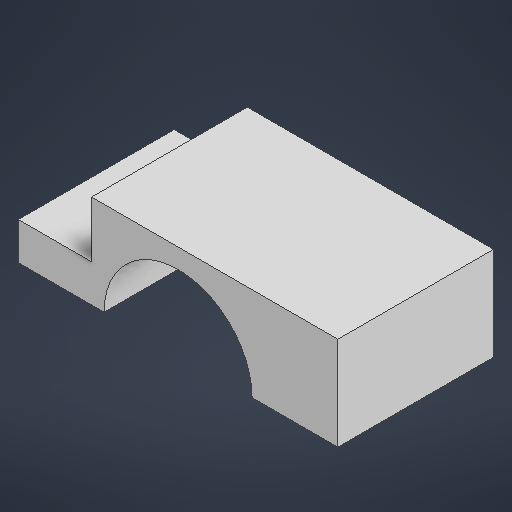
# Autodesk Inventor part: dg_clamp
Saved by Autodesk Inventor 2026.1 (Build 301233020, 233B)
## iProperties
Created: 2026-03-05
Part Number: dg_clamp
Material: Generic
Document SubType Name: Modeling
Designer: Dylan
Density: 1 g/cm^3
Appearance: Default
Author: Dylan
Autodesk Inventor part; units mm, degrees
ref_plane "YZ Plane" through (0, 0, 0) normal (1, 0, 0) x (0, 1, 0)
ref_plane "XZ Plane" through (0, 0, 0) normal (0, 1, 0) x (-1, 0, 0)
ref_plane "XY Plane" through (0, 0, 0) normal (0, 0, 1) x (1, 0, 0)
sketch "Sketch1" plane through (0, 0, 0) normal (0, 1, 0) x (-1, 0, 0)
  line L0 (0, 0) -> (-20.51, 0)
  line L1 (-20.51, 0) -> (-20.51, -10)
  line L2 (-20.51, -10) -> (0, -10)
  line L3 (0, -10) -> (0, 0)
  dimension "d0" = 20.51
  dimension "d1" = 10
  constraints: 8 end point, 2 parallel, 1 horizontal, 1 perpendicular
  measures "d0" distance of L2.end L1.end
  measures "d1" distance of L1.end L0.end
extrude "Extrusion1" add sketch "Sketch1" along normal blind 6
sketch "Sketch3" plane through (20.51, 0, -10) normal (0, 0, -1) x (-1, 0, 0)
  line L0 (0, 0) -> (20.51, 0) projected
  circle A0 centre (10.255, 0) radius 4.75
  point P0 (15.005, 0)
  point P1 (5.505, 0)
  dimension "d4" = 9.5
  constraints: 1 centre point, 1 midpoint
  measures "d4" diameter of A0
extrude "Extrusion2" cut sketch "Sketch3" against normal through all contours A0 L0 picked at (11.657, 0.7358)
sketch "Sketch7" plane through (0, 6, 0) normal (0, 1, 0) x (1, 0, 0)
  line L0 (0, 0) -> (20.51, 0) projected
  line L1 (20.51, 10) -> (0, 10) projected
  line L2 (4.7, 0) -> (0, 0)
  line L3 (0, 0) -> (0, 10)
  line L4 (0, 10) -> (4.7, 10)
  line L5 (4.7, 10) -> (4.7, 0)
  constraints: 8 end point, 2 parallel, 1 horizontal, 1 perpendicular, 1 point on line
extrude "Extrusion3" cut sketch "Sketch7" against normal blind 3.6
sketch "Sketch8" plane through (0, 2.4, 0) normal (0, 1, 0) x (1, 0, 0)
  circle A0 centre (3, 5) radius 1.075
  point P0 (0, 0)
  dimension "d9" = 2.15
  constraints: 1 centre point
  measures "d9" diameter of A0
extrude "Extrusion4" cut sketch "Sketch8" against normal through all
chamfer "Chamfer1" distance 0.4 angle 45 1 edges at (1.925, 2.4, -5)
body "Solid1"
